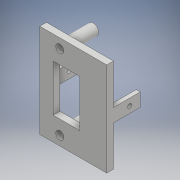
# Autodesk Inventor part: Support Poulie Bas
Saved by Autodesk Inventor 2017 (Build 210142000, 142)
## iProperties
Part Number: Support Poulie Bas
Material: Générique
Document SubType Name: Modeling
Designer: sasha
Density: 1 g/cm^3
Appearance: Par défaut
Author: sasha
Autodesk Inventor part; units mm, degrees
ref_plane "YZ Plane" through (0, 0, 0) normal (1, 0, 0) x (0, 1, 0)
ref_plane "XZ Plane" through (0, 0, 0) normal (0, 1, 0) x (-1, 0, 0)
ref_plane "XY Plane" through (0, 0, 0) normal (0, 0, 1) x (1, 0, 0)
sketch "Esquisse1" plane through (0, 0, 0) normal (0, 1, 0) x (-1, 0, 0)
  line L0 (0, 0) -> (50, 0)
  line L1 (50, 0) -> (50, -70)
  line L2 (50, -70) -> (0, -70)
  line L3 (0, -70) -> (0, 0)
  circle A0 centre (35, -7) radius 3
  circle A1 centre (35, -63) radius 3
  line L4 (35, -4) -> (35, -10)
  line L5 (35, -60) -> (35, -66)
  circle A2 centre (35, -7) radius 3
  circle A3 centre (35, -63) radius 3
  dimension "d0" = 70
  dimension "d1" = 50
  dimension "d3" = 7
  dimension "d4" = 7
  dimension "d5" = 6
  dimension "d6" = 6
  constraints: 12 end point, 4 centre point, 4 coincident, 4 point on circle, 3 perpendicular, 2 concentric, 2 midpoint, 2 parallel, 1 horizontal
  measures "d0" distance of L0.end L1.end
  measures "d1" distance of L1.end L2.end
  measures "d3" distance from line of L0 point (35, -7)
  measures "d4" distance from line of L2 point (35, -63)
  measures "d5" diameter of A0
  measures "d6" diameter of A1
extrude "Extrusion1" add sketch "Esquisse1" along normal blind 5
sketch "Esquisse2" plane through (0, 5, 0) normal (0, 1, 0) x (1, 0, 0)
  circle A0 centre (-35, 7) radius 3 projected
  circle A1 centre (-35, 7) radius 3
  circle A2 centre (-35, 63) radius 3 projected
  circle A3 centre (-35, 63) radius 3
  circle A4 centre (-35, 63) radius 4
  circle A5 centre (-35, 7) radius 4
  line L0 (0, 70) -> (-50, 70) projected
  line L1 (0, 0) -> (-3, 0)
  line L2 (-3, 30) -> (-3, 40)
  line L3 (-3, 70) -> (0, 70)
  line L4 (0, 70) -> (0, 0)
  line L5 (-50, 40) -> (-45, 40)
  line L6 (-45, 40) -> (-45, 30)
  line L7 (-45, 30) -> (-50, 30)
  line L8 (-50, 30) -> (-50, 40)
  line L9 (-50, 70) -> (-50, 0) projected
  line L10 (0, 0) -> (0, 70) projected
  line L11 (0, 40) -> (-3, 40)
  line L12 (0, 30) -> (-3, 30)
  line L13 (0, 40) -> (-3, 40)
  line L14 (-3, 40) -> (-3, 30)
  line L15 (-3, 30) -> (0, 30)
  line L16 (0, 30) -> (0, 40)
  point P0 (-50, 35)
  point P1 (-50, 35)
  dimension "d9" = 8
  dimension "d10" = 8
  dimension "d11" = 3
  dimension "d19" = 5
  dimension "d20" = 10
  constraints: 28 end point, 6 parallel, 5 perpendicular, 4 centre point, 4 coincident, 3 horizontal, 3 midpoint, 3 point on line, 2 collinear
  measures "d9" diameter of A4
  measures "d10" diameter of A5
  measures "d11" distance of L3.start L3.end
  measures "d19" distance of L5.start L5.end
  measures "d20" distance of L5.end L6.end
sketch "Esquisse3" plane through (0, 5, 0) normal (0, 1, 0) x (1, 0, 0)
  line L0 (-40, 52.5) -> (-20, 52.5)
  line L1 (-20, 52.5) -> (-20, 17.5)
  line L2 (-20, 17.5) -> (-40, 17.5)
  line L3 (-40, 17.5) -> (-40, 52.5)
  line L4 (-40, 35) -> (-20, 35)
  line L5 (-50, 70) -> (-50, 0) projected
  line L6 (-50, 35) -> (-3, 35)
  line L7 (-3, 70) -> (-3, 0) projected
  point P0 (0, 0)
  dimension "d14" = 35
  dimension "d15" = 20
  dimension "d16" = 10
  constraints: 12 end point, 4 midpoint, 2 parallel, 1 collinear, 1 horizontal, 1 perpendicular
  measures "d14" distance of L2.end L0.start
  measures "d15" distance of L0.start L0.end
  measures "d16" distance between parallel lines of L5 L3
extrude "Extrusion3" cut sketch "Esquisse3" against normal through all
extrude "Extrusion4" add sketch "Esquisse2" along normal blind 20
sketch "Esquisse5" plane through (0, 0, 0) normal (1, 0, 0) x (0, 0, -1)
  line L0 (17.5, 0) -> (52.5, 0) projected
  line L1 (35, 0) -> (35, 17)
  point P0 (0, 0)
  dimension "d23" = 17
  constraints: 2 end point, 1 coincident, 1 midpoint, 1 vertical
  measures "d23" distance of L1.start L1.end
hole "Perçage1" at (0, 17, -35) direction (-1, 0, 0) diameter 3 end through all
